Autodesk Fusion 360 part; units mm, degrees
(part 2 of 9)
  constraint tangent L185 A185
  constraint tangent L186 A185
  constraint equal A185 A186
  constraint tangent L186 A187
  constraint tangent L187 A187
  constraint equal A186 A187
  constraint horizontal L188
  constraint vertical L189
  constraint horizontal L190
  constraint vertical L191
  constraint tangent L188 A190
  constraint tangent L191 A190
  constraint tangent L188 A188
  constraint tangent L189 A188
  constraint equal A188 A190
  constraint tangent L189 A189
  constraint tangent L190 A189
  constraint equal A189 A190
  constraint tangent L190 A191
  constraint tangent L191 A191
  constraint equal A190 A191
  measures "d16" distance of L1 P0
  measures "d17" distance of L2 P0
  measures "d18" distance of P1 P2
  measures "d19" distance of P1 P3
  measures "d20" distance of P0 L11
  measures "d21" distance of P0 L8
  measures "d22" radius of A8
  measures "d23" distance of P0 P4
  measures "d24" radius of A13
  measures "d25" radius of A18
  measures "d26" radius of A22
  measures "d27" radius of A26
  measures "d28" radius of A30
  measures "d29" radius of A34
  measures "d30" radius of A38
  measures "d31" radius of A42
  measures "d32" radius of A46
  measures "d33" radius of A50
  measures "d34" radius of A54
  measures "d35" radius of A58
  measures "d36" radius of A62
  measures "d37" radius of A66
  measures "d38" radius of A70
  measures "d39" radius of A74
  measures "d40" radius of A78
  measures "d41" radius of A82
  measures "d42" radius of A86
  measures "d43" radius of A90
  measures "d44" radius of A94
  measures "d45" radius of A98
  measures "d46" radius of A102
  measures "d47" radius of A106
  measures "d48" radius of A110
  measures "d49" radius of A114
  measures "d50" radius of A118
  measures "d51" radius of A122
  measures "d52" radius of A126
  measures "d53" radius of A130
  measures "d54" radius of A134
  measures "d55" radius of A138
  measures "d56" radius of A142
  measures "d57" radius of A146
  measures "d58" radius of A150
  measures "d59" radius of A154
  measures "d60" radius of A158
  measures "d61" radius of A162
  measures "d62" radius of A166
  measures "d63" radius of A170
  measures "d64" radius of A174
  measures "d65" radius of A178
  measures "d66" radius of A182
  measures "d67" radius of A186
  measures "d68" radius of A190
extrude "Extrude3" cut sketch "Sketch3" against normal blind 5.1 contours L8 L9 L10 A9 A10 L188 L190 L191 A190 A191 | L9 A9 A10 L188 L189 L190 A188 A189 | A12 L12 A13 L13 A14 L14 L15 A15 | L16 L17 L18 L19 A16 A17 A18 A19 | L20 L21 L22 L23 A20 A21 A22 A23 | L24 L25 L26 L27 A24 A25 A26 A27 | L28 L29 L30 L31 A28 A29 A30 A31 | L32 L33 L34 L35 A32 A33 A34 A35 | L36 L37 L38 L39 A36 A37 A38 A39 | L40 L41 L42 L43 A40 A41 A42 A43 | L44 L45 L46 L47 A44 A45 A46 A47 | L48 L49 L50 L51 A48 A49 A50 A51 | L52 L53 L54 L55 A52 A53 A54 A55 | L56 L57 L58 L59 A56 A57 A58 A59 | L60 L61 L62 L63 A60 A61 A62 A63 | L64 L65 L66 L67 A64 A65 A66 A67 | L68 L69 L70 L71 A68 A69 A70 A71 | L72 L73 L74 L75 A72 A73 A74 A75 | L76 L77 L78 L79 A76 A77 A78 A79 | L80 L81 L82 L83 A80 A81 A82 A83 | L84 L85 L86 L87 A84 A85 A86 A87 | L88 L89 L90 L91 A88 A89 A90 A91 | L92 L93 L94 L95 A92 A93 A94 A95 | L96 L97 L98 L99 A96 A97 A98 A99 | L100 L101 L102 L103 A100 A101 A102 A103 | L104 L105 L106 L107 A104 A105 A106 A107 | L108 L109 L110 L111 A108 A109 A110 A111 | L112 L113 L114 L115 A112 A113 A114 A115 | L116 L117 L118 L119 A116 A117 A118 A119 | L120 L121 L122 L123 A120 A121 A122 A123 | L124 L125 L126 L127 A124 A125 A126 A127 | L128 L129 L130 L131 A128 A129 A130 A131 | L132 L133 L134 L135 A132 A133 A134 A135 | L136 L137 L138 L139 A136 A137 A138 A139 | L140 L141 L142 L143 A140 A141 A142 A143 | L144 L145 L146 L147 A144 A145 A146 A147 | L148 L149 L150 L151 A148 A149 A150 A151 | L152 L153 L154 L155 A152 A153 A154 A155 | L156 L157 L158 L159 A156 A157 A158 A159 | L160 L161 L162 L163 A160 A161 A162 A163 | L164 L165 L166 L167 A164 A165 A166 A167 | L168 L169 L170 L171 A168 A169 A170 A171 | L172 L173 L174 L175 A172 A173 A174 A175 | L176 L177 L178 L179 A176 A177 A178 A179 | L180 L181 L182 L183 A180 A181 A182 A183 | L184 L185 L186 L187 A184 A185 A186 A187
sketch "Sketch4" plane through (0, 5.1, 0) normal (0, 1, 0) x (-1, 0, 0)
  line L0 (-250.175, 15.525) -> (-250.175, 3.525)
  arc A0 (-251.175, 2.525) -> (-250.175, 3.525) centre (-251.175, 3.525) ccw
  line L1 (-251.175, 2.525) -> (-263.175, 2.525)
  arc A1 (-264.175, 3.525) -> (-263.175, 2.525) centre (-263.175, 3.525) ccw
  line L2 (-264.175, 3.525) -> (-264.175, 15.525)
  arc A2 (-263.175, 16.525) -> (-264.175, 15.525) centre (-263.175, 15.525) ccw
  line L3 (-263.175, 16.525) -> (-251.175, 16.525)
  arc A3 (-250.175, 15.525) -> (-251.175, 16.525) centre (-251.175, 15.525) ccw
  line L4 (-216.8375, 53.625) -> (-216.8375, 41.625)
  arc A4 (-217.8375, 40.625) -> (-216.8375, 41.625) centre (-217.8375, 41.625) ccw
  line L5 (-217.8375, 40.625) -> (-229.8375, 40.625)
  arc A5 (-230.8375, 41.625) -> (-229.8375, 40.625) centre (-229.8375, 41.625) ccw
  line L6 (-230.8375, 41.625) -> (-230.8375, 53.625)
  arc A6 (-229.8375, 54.625) -> (-230.8375, 53.625) centre (-229.8375, 53.625) ccw
  line L7 (-229.8375, 54.625) -> (-217.8375, 54.625)
  arc A7 (-216.8375, 53.625) -> (-217.8375, 54.625) centre (-217.8375, 53.625) ccw
  line L8 (-188.2625, 34.575) -> (-188.2625, 22.575)
  arc A8 (-189.2625, 21.575) -> (-188.2625, 22.575) centre (-189.2625, 22.575) ccw
  line L9 (-189.2625, 21.575) -> (-201.2625, 21.575)
  arc A9 (-202.2625, 22.575) -> (-201.2625, 21.575) centre (-201.2625, 22.575) ccw
  line L10 (-202.2625, 22.575) -> (-202.2625, 34.575)
  arc A10 (-201.2625, 35.575) -> (-202.2625, 34.575) centre (-201.2625, 34.575) ccw
  line L11 (-201.2625, 35.575) -> (-189.2625, 35.575)
  arc A11 (-188.2625, 34.575) -> (-189.2625, 35.575) centre (-189.2625, 34.575) ccw
  line L12 (-178.7375, 53.625) -> (-178.7375, 41.625)
  arc A12 (-179.7375, 40.625) -> (-178.7375, 41.625) centre (-179.7375, 41.625) ccw
  line L13 (-179.7375, 40.625) -> (-191.7375, 40.625)
  arc A13 (-192.7375, 41.625) -> (-191.7375, 40.625) centre (-191.7375, 41.625) ccw
  line L14 (-192.7375, 41.625) -> (-192.7375, 53.625)
  arc A14 (-191.7375, 54.625) -> (-192.7375, 53.625) centre (-191.7375, 53.625) ccw
  line L15 (-191.7375, 54.625) -> (-179.7375, 54.625)
  arc A15 (-178.7375, 53.625) -> (-179.7375, 54.625) centre (-179.7375, 53.625) ccw
  line L16 (-140.6375, 53.625) -> (-140.6375, 41.625)
  arc A16 (-141.6375, 40.625) -> (-140.6375, 41.625) centre (-141.6375, 41.625) ccw
  line L17 (-141.6375, 40.625) -> (-153.6375, 40.625)
  arc A17 (-154.6375, 41.625) -> (-153.6375, 40.625) centre (-153.6375, 41.625) ccw
  line L18 (-154.6375, 41.625) -> (-154.6375, 53.625)
  arc A18 (-153.6375, 54.625) -> (-154.6375, 53.625) centre (-153.6375, 53.625) ccw
  line L19 (-153.6375, 54.625) -> (-141.6375, 54.625)
  arc A19 (-140.6375, 53.625) -> (-141.6375, 54.625) centre (-141.6375, 53.625) ccw
  line L20 (-131.1125, 34.575) -> (-131.1125, 22.575)
  arc A20 (-132.1125, 21.575) -> (-131.1125, 22.575) centre (-132.1125, 22.575) ccw
  line L21 (-132.1125, 21.575) -> (-144.1125, 21.575)
  arc A21 (-145.1125, 22.575) -> (-144.1125, 21.575) centre (-144.1125, 22.575) ccw
  line L22 (-145.1125, 22.575) -> (-145.1125, 34.575)
  arc A22 (-144.1125, 35.575) -> (-145.1125, 34.575) centre (-144.1125, 34.575) ccw
  line L23 (-144.1125, 35.575) -> (-132.1125, 35.575)
  arc A23 (-131.1125, 34.575) -> (-132.1125, 35.575) centre (-132.1125, 34.575) ccw
  line L24 (-107.3, 15.525) -> (-107.3, 3.525)
  arc A24 (-108.3, 2.525) -> (-107.3, 3.525) centre (-108.3, 3.525) ccw
  line L25 (-108.3, 2.525) -> (-120.3, 2.525)
  arc A25 (-121.3, 3.525) -> (-120.3, 2.525) centre (-120.3, 3.525) ccw
  line L26 (-121.3, 3.525) -> (-121.3, 15.525)
  arc A26 (-120.3, 16.525) -> (-121.3, 15.525) centre (-120.3, 15.525) ccw
  line L27 (-120.3, 16.525) -> (-108.3, 16.525)
  arc A27 (-107.3, 15.525) -> (-108.3, 16.525) centre (-108.3, 15.525) ccw
  line L28 (-100.1562, 72.675) -> (-100.1562, 60.675)
  arc A28 (-101.1563, 59.675) -> (-100.1562, 60.675) centre (-101.1562, 60.675) ccw
  line L29 (-101.1563, 59.675) -> (-113.1562, 59.675)
  arc A29 (-114.1562, 60.675) -> (-113.1562, 59.675) centre (-113.1562, 60.675) ccw
  line L30 (-114.1562, 60.675) -> (-114.1562, 72.675)
  arc A30 (-113.1562, 73.675) -> (-114.1562, 72.675) centre (-113.1562, 72.675) ccw
  line L31 (-113.1562, 73.675) -> (-101.1562, 73.675)
  arc A31 (-100.1562, 72.675) -> (-101.1563, 73.675) centre (-101.1562, 72.675) ccw
  line L32 (-69.2, 15.525) -> (-69.2, 3.525)
  arc A32 (-70.2, 2.525) -> (-69.2, 3.525) centre (-70.2, 3.525) ccw
  line L33 (-70.2, 2.525) -> (-82.2, 2.525)
  arc A33 (-83.2, 3.525) -> (-82.2, 2.525) centre (-82.2, 3.525) ccw
  line L34 (-83.2, 3.525) -> (-83.2, 15.525)
  arc A34 (-82.2, 16.525) -> (-83.2, 15.525) centre (-82.2, 15.525) ccw
  line L35 (-82.2, 16.525) -> (-70.2, 16.525)
  arc A35 (-69.2, 15.525) -> (-70.2, 16.525) centre (-70.2, 15.525) ccw
  line L36 (-45.3875, 53.625) -> (-45.3875, 41.625)
  arc A36 (-46.3875, 40.625) -> (-45.3875, 41.625) centre (-46.3875, 41.625) ccw
  line L37 (-46.3875, 40.625) -> (-58.3875, 40.625)
  arc A37 (-59.3875, 41.625) -> (-58.3875, 40.625) centre (-58.3875, 41.625) ccw
  line L38 (-59.3875, 41.625) -> (-59.3875, 53.625)
  arc A38 (-58.3875, 54.625) -> (-59.3875, 53.625) centre (-58.3875, 53.625) ccw
  line L39 (-58.3875, 54.625) -> (-46.3875, 54.625)
  arc A39 (-45.3875, 53.625) -> (-46.3875, 54.625) centre (-46.3875, 53.625) ccw
  line L40 (-9.6688, 34.575) -> (-9.6687, 22.575)
  arc A40 (-10.6687, 21.575) -> (-9.6687, 22.575) centre (-10.6688, 22.575) ccw
  line L41 (-10.6687, 21.575) -> (-22.6688, 21.575)
  arc A41 (-23.6688, 22.575) -> (-22.6688, 21.575) centre (-22.6687, 22.575) ccw
  line L42 (-23.6688, 22.575) -> (-23.6687, 34.575)
  arc A42 (-22.6687, 35.575) -> (-23.6687, 34.575) centre (-22.6687, 34.575) ccw
  line L43 (-22.6688, 35.575) -> (-10.6688, 35.575)
  arc A43 (-9.6688, 34.575) -> (-10.6687, 35.575) centre (-10.6688, 34.575) ccw
  line L44 (-44.1, 16.525) -> (-32.1, 16.525)
  arc A44 (-31.1, 15.525) -> (-32.1, 16.525) centre (-32.1, 15.525) ccw
  line L45 (-31.1, 15.525) -> (-31.1, 3.525)
  arc A45 (-32.1, 2.525) -> (-31.1, 3.525) centre (-32.1, 3.525) ccw
  line L46 (-32.1, 2.525) -> (-44.1, 2.525)
  arc A46 (-45.1, 3.525) -> (-44.1, 2.525) centre (-44.1, 3.525) ccw
  line L47 (-45.1, 3.525) -> (-45.1, 15.525)
  arc A47 (-44.1, 16.525) -> (-45.1, 15.525) centre (-44.1, 15.525) ccw
  line L48 (-40.625, 72.675) -> (-40.625, 60.675)
  arc A48 (-41.625, 59.675) -> (-40.625, 60.675) centre (-41.625, 60.675) ccw
  line L49 (-41.625, 59.675) -> (-53.625, 59.675)
  arc A49 (-54.625, 60.675) -> (-53.625, 59.675) centre (-53.625, 60.675) ccw
  line L50 (-54.625, 60.675) -> (-54.625, 72.675)
  arc A50 (-53.625, 73.675) -> (-54.625, 72.675) centre (-53.625, 72.675) ccw
  line L51 (-53.625, 73.675) -> (-41.625, 73.675)
  arc A51 (-40.625, 72.675) -> (-41.625, 73.675) centre (-41.625, 72.675) ccw
  line L52 (-54.9125, 34.575) -> (-54.9125, 22.575)
  arc A52 (-55.9125, 21.575) -> (-54.9125, 22.575) centre (-55.9125, 22.575) ccw
  line L53 (-55.9125, 21.575) -> (-67.9125, 21.575)
  arc A53 (-68.9125, 22.575) -> (-67.9125, 21.575) centre (-67.9125, 22.575) ccw
  line L54 (-68.9125, 22.575) -> (-68.9125, 34.575)
  arc A54 (-67.9125, 35.575) -> (-68.9125, 34.575) centre (-67.9125, 34.575) ccw
  line L55 (-67.9125, 35.575) -> (-55.9125, 35.575)
  arc A55 (-54.9125, 34.575) -> (-55.9125, 35.575) centre (-55.9125, 34.575) ccw
  line L56 (-66.8188, 72.675) -> (-66.8188, 60.675)
  arc A56 (-67.8188, 59.675) -> (-66.8188, 60.675) centre (-67.8188, 60.675) ccw
  line L57 (-67.8188, 59.675) -> (-79.8188, 59.675)
  arc A57 (-80.8188, 60.675) -> (-79.8188, 59.675) centre (-79.8188, 60.675) ccw
  line L58 (-80.8187, 60.675) -> (-80.8187, 72.675)
  arc A58 (-79.8188, 73.675) -> (-80.8188, 72.675) centre (-79.8188, 72.675) ccw
  line L59 (-79.8188, 73.675) -> (-67.8188, 73.675)
  arc A59 (-66.8188, 72.675) -> (-67.8188, 73.675) centre (-67.8188, 72.675) ccw
  line L60 (-88.25, 15.525) -> (-88.25, 3.525)
  arc A60 (-89.25, 2.525) -> (-88.25, 3.525) centre (-89.25, 3.525) ccw
  line L61 (-89.25, 2.525) -> (-101.25, 2.525)
  arc A61 (-102.25, 3.525) -> (-101.25, 2.525) centre (-101.25, 3.525) ccw
  line L62 (-102.25, 3.525) -> (-102.25, 15.525)
  arc A62 (-101.25, 16.525) -> (-102.25, 15.525) centre (-101.25, 15.525) ccw
  line L63 (-101.25, 16.525) -> (-89.25, 16.525)
  arc A63 (-88.25, 15.525) -> (-89.25, 16.525) centre (-89.25, 15.525) ccw
  line L64 (-121.5875, 53.625) -> (-121.5875, 41.625)
  arc A64 (-122.5875, 40.625) -> (-121.5875, 41.625) centre (-122.5875, 41.625) ccw
  line L65 (-122.5875, 40.625) -> (-134.5875, 40.625)
  arc A65 (-135.5875, 41.625) -> (-134.5875, 40.625) centre (-134.5875, 41.625) ccw
  line L66 (-135.5875, 41.625) -> (-135.5875, 53.625)
  arc A66 (-134.5875, 54.625) -> (-135.5875, 53.625) centre (-134.5875, 53.625) ccw
  line L67 (-134.5875, 54.625) -> (-122.5875, 54.625)
  arc A67 (-121.5875, 53.625) -> (-122.5875, 54.625) centre (-122.5875, 53.625) ccw
  line L68 (-150.1625, 34.575) -> (-150.1625, 22.575)
  arc A68 (-151.1625, 21.575) -> (-150.1625, 22.575) centre (-151.1625, 22.575) ccw
  line L69 (-151.1625, 21.575) -> (-163.1625, 21.575)
  arc A69 (-164.1625, 22.575) -> (-163.1625, 21.575) centre (-163.1625, 22.575) ccw
  line L70 (-164.1625, 22.575) -> (-164.1625, 34.575)
  arc A70 (-163.1625, 35.575) -> (-164.1625, 34.575) centre (-163.1625, 34.575) ccw
  line L71 (-163.1625, 35.575) -> (-151.1625, 35.575)
  arc A71 (-150.1625, 34.575) -> (-151.1625, 35.575) centre (-151.1625, 34.575) ccw
  line L72 (-171.5938, 72.675) -> (-171.5937, 60.675)
  arc A72 (-172.5937, 59.675) -> (-171.5937, 60.675) centre (-172.5937, 60.675) ccw
  line L73 (-172.5938, 59.675) -> (-184.5938, 59.675)
  arc A73 (-185.5938, 60.675) -> (-184.5938, 59.675) centre (-184.5938, 60.675) ccw
  line L74 (-185.5938, 60.675) -> (-185.5937, 72.675)
  arc A74 (-184.5938, 73.675) -> (-185.5937, 72.675) centre (-184.5937, 72.675) ccw
  line L75 (-184.5938, 73.675) -> (-172.5937, 73.675)
  arc A75 (-171.5938, 72.675) -> (-172.5937, 73.675) centre (-172.5937, 72.675) ccw
  line L76 (-183.5, 15.525) -> (-183.5, 3.525)
  arc A76 (-184.5, 2.525) -> (-183.5, 3.525) centre (-184.5, 3.525) ccw
  line L77 (-184.5, 2.525) -> (-196.5, 2.525)
  arc A77 (-197.5, 3.525) -> (-196.5, 2.525) centre (-196.5, 3.525) ccw
  line L78 (-197.5, 3.525) -> (-197.5, 15.525)
  arc A78 (-196.5, 16.525) -> (-197.5, 15.525) centre (-196.5, 15.525) ccw
  line L79 (-196.5, 16.525) -> (-184.5, 16.525)
  arc A79 (-183.5, 15.525) -> (-184.5, 16.525) centre (-184.5, 15.525) ccw
  line L80 (-223.9813, 72.675) -> (-223.9813, 60.675)
  arc A80 (-224.9813, 59.675) -> (-223.9812, 60.675) centre (-224.9812, 60.675) ccw
  line L81 (-224.9813, 59.675) -> (-236.9813, 59.675)
  arc A81 (-237.9813, 60.675) -> (-236.9813, 59.675) centre (-236.9813, 60.675) ccw
  line L82 (-237.9813, 60.675) -> (-237.9812, 72.675)
  arc A82 (-236.9813, 73.675) -> (-237.9813, 72.675) centre (-236.9813, 72.675) ccw
  line L83 (-236.9813, 73.675) -> (-224.9813, 73.675)
  arc A83 (-223.9813, 72.675) -> (-224.9813, 73.675) centre (-224.9812, 72.675) ccw
  line L84 (-226.3625, 15.525) -> (-226.3625, 3.525)
  arc A84 (-227.3625, 2.525) -> (-226.3625, 3.525) centre (-227.3625, 3.525) ccw
  line L85 (-227.3625, 2.525) -> (-239.3625, 2.525)
  arc A85 (-240.3625, 3.525) -> (-239.3625, 2.525) centre (-239.3625, 3.525) ccw
  line L86 (-240.3625, 3.525) -> (-240.3625, 15.525)
  arc A86 (-239.3625, 16.525) -> (-240.3625, 15.525) centre (-239.3625, 15.525) ccw
  line L87 (-239.3625, 16.525) -> (-227.3625, 16.525)
  arc A87 (-226.3625, 15.525) -> (-227.3625, 16.525) centre (-227.3625, 15.525) ccw
  line L88 (-238.2688, 34.575) -> (-238.2688, 22.575)
  arc A88 (-239.2688, 21.575) -> (-238.2687, 22.575) centre (-239.2687, 22.575) ccw
  line L89 (-239.2688, 21.575) -> (-251.2688, 21.575)
  arc A89 (-252.2688, 22.575) -> (-251.2688, 21.575) centre (-251.2688, 22.575) ccw
  line L90 (-252.2688, 22.575) -> (-252.2688, 34.575)
  arc A90 (-251.2688, 35.575) -> (-252.2688, 34.575) centre (-251.2687, 34.575) ccw
  line L91 (-251.2688, 35.575) -> (-239.2688, 35.575)
  arc A91 (-238.2688, 34.575) -> (-239.2688, 35.575) centre (-239.2687, 34.575) ccw
  line L92 (-207.3125, 34.575) -> (-207.3125, 22.575)
  arc A92 (-208.3125, 21.575) -> (-207.3125, 22.575) centre (-208.3125, 22.575) ccw
  line L93 (-208.3125, 21.575) -> (-220.3125, 21.575)
  arc A93 (-221.3125, 22.575) -> (-220.3125, 21.575) centre (-220.3125, 22.575) ccw
  line L94 (-221.3125, 22.575) -> (-221.3125, 34.575)
  arc A94 (-220.3125, 35.575) -> (-221.3125, 34.575) centre (-220.3125, 34.575) ccw
  line L95 (-220.3125, 35.575) -> (-208.3125, 35.575)
  arc A95 (-207.3125, 34.575) -> (-208.3125, 35.575) centre (-208.3125, 34.575) ccw
  line L96 (-197.7875, 53.625) -> (-197.7875, 41.625)
  arc A96 (-198.7875, 40.625) -> (-197.7875, 41.625) centre (-198.7875, 41.625) ccw
  line L97 (-198.7875, 40.625) -> (-210.7875, 40.625)
  arc A97 (-211.7875, 41.625) -> (-210.7875, 40.625) centre (-210.7875, 41.625) ccw
  line L98 (-211.7875, 41.625) -> (-211.7875, 53.625)
  arc A98 (-210.7875, 54.625) -> (-211.7875, 53.625) centre (-210.7875, 53.625) ccw
  line L99 (-210.7875, 54.625) -> (-198.7875, 54.625)
  arc A99 (-197.7875, 53.625) -> (-198.7875, 54.625) centre (-198.7875, 53.625) ccw
  line L100 (-169.2125, 34.575) -> (-169.2125, 22.575)
  arc A100 (-170.2125, 21.575) -> (-169.2125, 22.575) centre (-170.2125, 22.575) ccw
  line L101 (-170.2125, 21.575) -> (-182.2125, 21.575)
  arc A101 (-183.2125, 22.575) -> (-182.2125, 21.575) centre (-182.2125, 22.575) ccw
  line L102 (-183.2125, 22.575) -> (-183.2125, 34.575)
  arc A102 (-182.2125, 35.575) -> (-183.2125, 34.575) centre (-182.2125, 34.575) ccw
  line L103 (-182.2125, 35.575) -> (-170.2125, 35.575)
  arc A103 (-169.2125, 34.575) -> (-170.2125, 35.575) centre (-170.2125, 34.575) ccw
  line L104 (-140.6375, 72.675) -> (-140.6375, 60.675)
  arc A104 (-141.6375, 59.675) -> (-140.6375, 60.675) centre (-141.6375, 60.675) ccw
  line L105 (-141.6375, 59.675) -> (-153.6375, 59.675)
  arc A105 (-154.6375, 60.675) -> (-153.6375, 59.675) centre (-153.6375, 60.675) ccw
  line L106 (-154.6375, 60.675) -> (-154.6375, 72.675)
  arc A106 (-153.6375, 73.675) -> (-154.6375, 72.675) centre (-153.6375, 72.675) ccw
  line L107 (-153.6375, 73.675) -> (-141.6375, 73.675)
  arc A107 (-140.6375, 72.675) -> (-141.6375, 73.675) centre (-141.6375, 72.675) ccw
  line L108 (-126.35, 15.525) -> (-126.35, 3.525)
  arc A108 (-127.35, 2.525) -> (-126.35, 3.525) centre (-127.35, 3.525) ccw
  line L109 (-127.35, 2.525) -> (-139.35, 2.525)
  arc A109 (-140.35, 3.525) -> (-139.35, 2.525) centre (-139.35, 3.525) ccw
  line L110 (-140.35, 3.525) -> (-140.35, 15.525)
  arc A110 (-139.35, 16.525) -> (-140.35, 15.525) centre (-139.35, 15.525) ccw
  line L111 (-139.35, 16.525) -> (-127.35, 16.525)
  arc A111 (-126.35, 15.525) -> (-127.35, 16.525) centre (-127.35, 15.525) ccw
  line L112 (-112.0625, 34.575) -> (-112.0625, 22.575)
  arc A112 (-113.0625, 21.575) -> (-112.0625, 22.575) centre (-113.0625, 22.575) ccw
  line L113 (-113.0625, 21.575) -> (-125.0625, 21.575)
  arc A113 (-126.0625, 22.575) -> (-125.0625, 21.575) centre (-125.0625, 22.575) ccw
  line L114 (-126.0625, 22.575) -> (-126.0625, 34.575)
  arc A114 (-125.0625, 35.575) -> (-126.0625, 34.575) centre (-125.0625, 34.575) ccw
  line L115 (-125.0625, 35.575) -> (-113.0625, 35.575)
  arc A115 (-112.0625, 34.575) -> (-113.0625, 35.575) centre (-113.0625, 34.575) ccw
  line L116 (-83.4875, 53.625) -> (-83.4875, 41.625)
  arc A116 (-84.4875, 40.625) -> (-83.4875, 41.625) centre (-84.4875, 41.625) ccw
  line L117 (-84.4875, 40.625) -> (-96.4875, 40.625)
  arc A117 (-97.4875, 41.625) -> (-96.4875, 40.625) centre (-96.4875, 41.625) ccw
  line L118 (-97.4875, 41.625) -> (-97.4875, 53.625)
  arc A118 (-96.4875, 54.625) -> (-97.4875, 53.625) centre (-96.4875, 53.625) ccw
  line L119 (-96.4875, 54.625) -> (-84.4875, 54.625)
  arc A119 (-83.4875, 53.625) -> (-84.4875, 54.625) centre (-84.4875, 53.625) ccw
  line L120 (-73.9625, 34.575) -> (-73.9625, 22.575)
  arc A120 (-74.9625, 21.575) -> (-73.9625, 22.575) centre (-74.9625, 22.575) ccw
  line L121 (-74.9625, 21.575) -> (-86.9625, 21.575)
  arc A121 (-87.9625, 22.575) -> (-86.9625, 21.575) centre (-86.9625, 22.575) ccw
  line L122 (-87.9625, 22.575) -> (-87.9625, 34.575)
  arc A122 (-86.9625, 35.575) -> (-87.9625, 34.575) centre (-86.9625, 34.575) ccw
  line L123 (-86.9625, 35.575) -> (-74.9625, 35.575)
  arc A123 (-73.9625, 34.575) -> (-74.9625, 35.575) centre (-74.9625, 34.575) ccw
  line L124 (-35.8625, 34.575) -> (-35.8625, 22.575)
  arc A124 (-36.8625, 21.575) -> (-35.8625, 22.575) centre (-36.8625, 22.575) ccw
  line L125 (-36.8625, 21.575) -> (-48.8625, 21.575)
  arc A125 (-49.8625, 22.575) -> (-48.8625, 21.575) centre (-48.8625, 22.575) ccw
  line L126 (-49.8625, 22.575) -> (-49.8625, 34.575)
  arc A126 (-48.8625, 35.575) -> (-49.8625, 34.575) centre (-48.8625, 34.575) ccw
  line L127 (-48.8625, 35.575) -> (-36.8625, 35.575)
  arc A127 (-35.8625, 34.575) -> (-36.8625, 35.575) centre (-36.8625, 34.575) ccw
  line L128 (-14.4313, 53.625) -> (-14.4313, 41.625)
  arc A128 (-15.4313, 40.625) -> (-14.4313, 41.625) centre (-15.4312, 41.625) ccw
  line L129 (-15.4313, 40.625) -> (-27.4313, 40.625)
  arc A129 (-28.4313, 41.625) -> (-27.4313, 40.625) centre (-27.4313, 41.625) ccw
  line L130 (-28.4313, 41.625) -> (-28.4313, 53.625)
  arc A130 (-27.4313, 54.625) -> (-28.4313, 53.625) centre (-27.4312, 53.625) ccw
  line L131 (-27.4313, 54.625) -> (-15.4313, 54.625)
  arc A131 (-14.4313, 53.625) -> (-15.4313, 54.625) centre (-15.4313, 53.625) ccw
  line L132 (-7.2875, 15.525) -> (-7.2875, 3.525)
  arc A132 (-8.2875, 2.525) -> (-7.2875, 3.525) centre (-8.2875, 3.525) ccw
  line L133 (-8.2875, 2.525) -> (-20.2875, 2.525)
  arc A133 (-21.2875, 3.525) -> (-20.2875, 2.525) centre (-20.2875, 3.525) ccw
  line L134 (-21.2875, 3.525) -> (-21.2875, 15.525)
  arc A134 (-20.2875, 16.525) -> (-21.2875, 15.525) centre (-20.2875, 15.525) ccw
  line L135 (-20.2875, 16.525) -> (-8.2875, 16.525)
  arc A135 (-7.2875, 15.525) -> (-8.2875, 16.525) centre (-8.2875, 15.525) ccw
  line L136 (-14.4313, 72.675) -> (-14.4313, 60.675)
  arc A136 (-15.4313, 59.675) -> (-14.4313, 60.675) centre (-15.4312, 60.675) ccw
  line L137 (-15.4313, 59.675) -> (-27.4313, 59.675)
  arc A137 (-28.4313, 60.675) -> (-27.4313, 59.675) centre (-27.4313, 60.675) ccw
  line L138 (-28.4313, 60.675) -> (-28.4312, 72.675)
  arc A138 (-27.4313, 73.675) -> (-28.4312, 72.675) centre (-27.4312, 72.675) ccw
  line L139 (-27.4313, 73.675) -> (-15.4313, 73.675)
  arc A139 (-14.4313, 72.675) -> (-15.4313, 73.675) centre (-15.4313, 72.675) ccw
  line L140 (-50.15, 15.525) -> (-50.15, 3.525)
  arc A140 (-51.15, 2.525) -> (-50.15, 3.525) centre (-51.15, 3.525) ccw
  line L141 (-51.15, 2.525) -> (-63.15, 2.525)
  arc A141 (-64.15, 3.525) -> (-63.15, 2.525) centre (-63.15, 3.525) ccw
  line L142 (-64.15, 3.525) -> (-64.15, 15.525)
  arc A142 (-63.15, 16.525) -> (-64.15, 15.525) centre (-63.15, 15.525) ccw
  line L143 (-63.15, 16.525) -> (-51.15, 16.525)
  arc A143 (-50.15, 15.525) -> (-51.15, 16.525) centre (-51.15, 15.525) ccw
  line L144 (-64.4375, 53.625) -> (-64.4375, 41.625)
  arc A144 (-65.4375, 40.625) -> (-64.4375, 41.625) centre (-65.4375, 41.625) ccw
  line L145 (-65.4375, 40.625) -> (-77.4375, 40.625)
  arc A145 (-78.4375, 41.625) -> (-77.4375, 40.625) centre (-77.4375, 41.625) ccw
  line L146 (-78.4375, 41.625) -> (-78.4375, 53.625)
  arc A146 (-77.4375, 54.625) -> (-78.4375, 53.625) centre (-77.4375, 53.625) ccw
  line L147 (-77.4375, 54.625) -> (-65.4375, 54.625)
  arc A147 (-64.4375, 53.625) -> (-65.4375, 54.625) centre (-65.4375, 53.625) ccw
  line L148 (-93.0125, 34.575) -> (-93.0125, 22.575)
  arc A148 (-94.0125, 21.575) -> (-93.0125, 22.575) centre (-94.0125, 22.575) ccw
  line L149 (-94.0125, 21.575) -> (-106.0125, 21.575)
  arc A149 (-107.0125, 22.575) -> (-106.0125, 21.575) centre (-106.0125, 22.575) ccw
  line L150 (-107.0125, 22.575) -> (-107.0125, 34.575)
  arc A150 (-106.0125, 35.575) -> (-107.0125, 34.575) centre (-106.0125, 34.575) ccw
  line L151 (-106.0125, 35.575) -> (-94.0125, 35.575)
  arc A151 (-93.0125, 34.575) -> (-94.0125, 35.575) centre (-94.0125, 34.575) ccw
  line L152 (-102.5375, 53.625) -> (-102.5375, 41.625)
  arc A152 (-103.5375, 40.625) -> (-102.5375, 41.625) centre (-103.5375, 41.625) ccw
  line L153 (-103.5375, 40.625) -> (-115.5375, 40.625)
  arc A153 (-116.5375, 41.625) -> (-115.5375, 40.625) centre (-115.5375, 41.625) ccw
  line L154 (-116.5375, 41.625) -> (-116.5375, 53.625)
  arc A154 (-115.5375, 54.625) -> (-116.5375, 53.625) centre (-115.5375, 53.625) ccw
  line L155 (-115.5375, 54.625) -> (-103.5375, 54.625)
  arc A155 (-102.5375, 53.625) -> (-103.5375, 54.625) centre (-103.5375, 53.625) ccw
  line L156 (-145.4, 15.525) -> (-145.4, 3.525)
  arc A156 (-146.4, 2.525) -> (-145.4, 3.525) centre (-146.4, 3.525) ccw
  line L157 (-146.4, 2.525) -> (-158.4, 2.525)
  arc A157 (-159.4, 3.525) -> (-158.4, 2.525) centre (-158.4, 3.525) ccw
  line L158 (-159.4, 3.525) -> (-159.4, 15.525)
  arc A158 (-158.4, 16.525) -> (-159.4, 15.525) centre (-158.4, 15.525) ccw
  line L159 (-158.4, 16.525) -> (-146.4, 16.525)
  arc A159 (-145.4, 15.525) -> (-146.4, 16.525) centre (-146.4, 15.525) ccw
  line L160 (-159.6875, 53.625) -> (-159.6875, 41.625)
  arc A160 (-160.6875, 40.625) -> (-159.6875, 41.625) centre (-160.6875, 41.625) ccw
  line L161 (-160.6875, 40.625) -> (-172.6875, 40.625)
  arc A161 (-173.6875, 41.625) -> (-172.6875, 40.625) centre (-172.6875, 41.625) ccw
  line L162 (-173.6875, 41.625) -> (-173.6875, 53.625)
  arc A162 (-172.6875, 54.625) -> (-173.6875, 53.625) centre (-172.6875, 53.625) ccw
  line L163 (-172.6875, 54.625) -> (-160.6875, 54.625)
  arc A163 (-159.6875, 53.625) -> (-160.6875, 54.625) centre (-160.6875, 53.625) ccw
  line L164 (-164.45, 15.525) -> (-164.45, 3.525)
  arc A164 (-165.45, 2.525) -> (-164.45, 3.525) centre (-165.45, 3.525) ccw
  line L165 (-165.45, 2.525) -> (-177.45, 2.525)
  arc A165 (-178.45, 3.525) -> (-177.45, 2.525) centre (-177.45, 3.525) ccw
  line L166 (-178.45, 3.525) -> (-178.45, 15.525)
  arc A166 (-177.45, 16.525) -> (-178.45, 15.525) centre (-177.45, 15.525) ccw
  line L167 (-177.45, 16.525) -> (-165.45, 16.525)
  arc A167 (-164.45, 15.525) -> (-165.45, 16.525) centre (-165.45, 15.525) ccw
  line L168 (-197.7875, 72.675) -> (-197.7875, 60.675)
  arc A168 (-198.7875, 59.675) -> (-197.7875, 60.675) centre (-198.7875, 60.675) ccw
  line L169 (-198.7875, 59.675) -> (-210.7875, 59.675)
  arc A169 (-211.7875, 60.675) -> (-210.7875, 59.675) centre (-210.7875, 60.675) ccw
  line L170 (-211.7875, 60.675) -> (-211.7875, 72.675)
  arc A170 (-210.7875, 73.675) -> (-211.7875, 72.675) centre (-210.7875, 72.675) ccw
  line L171 (-210.7875, 73.675) -> (-198.7875, 73.675)
  arc A171 (-197.7875, 72.675) -> (-198.7875, 73.675) centre (-198.7875, 72.675) ccw
  line L172 (-202.55, 15.525) -> (-202.55, 3.525)
  arc A172 (-203.55, 2.525) -> (-202.55, 3.525) centre (-203.55, 3.525) ccw
  line L173 (-203.55, 2.525) -> (-215.55, 2.525)
  arc A173 (-216.55, 3.525) -> (-215.55, 2.525) centre (-215.55, 3.525) ccw
  line L174 (-216.55, 3.525) -> (-216.55, 15.525)
  arc A174 (-215.55, 16.525) -> (-216.55, 15.525) centre (-215.55, 15.525) ccw
  line L175 (-215.55, 16.525) -> (-203.55, 16.525)
  arc A175 (-202.55, 15.525) -> (-203.55, 16.525) centre (-203.55, 15.525) ccw
  line L176 (-243.0312, 53.625) -> (-243.0312, 41.625)
  arc A176 (-244.0312, 40.625) -> (-243.0313, 41.625) centre (-244.0313, 41.625) ccw
  line L177 (-244.0312, 40.625) -> (-256.0312, 40.625)
  arc A177 (-257.0312, 41.625) -> (-256.0312, 40.625) centre (-256.0312, 41.625) ccw
  line L178 (-257.0312, 41.625) -> (-257.0312, 53.625)
  arc A178 (-256.0312, 54.625) -> (-257.0312, 53.625) centre (-256.0312, 53.625) ccw
  line L179 (-256.0312, 54.625) -> (-244.0312, 54.625)
  arc A179 (-243.0313, 53.625) -> (-244.0312, 54.625) centre (-244.0312, 53.625) ccw
  arc A180 (-263.7, 57.15) -> (-266.7, 54.15) centre (-263.7, 54.15) ccw
  line L180 (-266.7, 54.15) -> (-266.7, 3)
  arc A181 (-266.7, 3) -> (-263.7, 0) centre (-263.7, 3) ccw
  line L181 (-263.7, 0) -> (-3, 0)
  arc A182 (-3, 0) -> (0, 3) centre (-3, 3) ccw
  line L182 (0, 3) -> (0, 54.15)
  arc A183 (0, 54.15) -> (-3, 57.15) centre (-3, 54.15) ccw
  line L183 (-3, 57.15) -> (-8.525, 57.15)
  arc A184 (-9.525, 58.15) -> (-8.525, 57.15) centre (-8.525, 58.15) ccw
  line L184 (-9.525, 58.15) -> (-9.525, 73.2)
  arc A185 (-9.525, 73.2) -> (-12.525, 76.2) centre (-12.525, 73.2) ccw
  line L185 (-12.525, 76.2) -> (-239.8875, 76.2)
  arc A186 (-239.8875, 76.2) -> (-242.8875, 73.2) centre (-239.8875, 73.2) ccw
  line L186 (-242.8875, 73.2) -> (-242.8875, 58.15)
  arc A187 (-243.8875, 57.15) -> (-242.8875, 58.15) centre (-243.8875, 58.15) ccw
  line L187 (-243.8875, 57.15) -> (-263.7, 57.15)
  line L188 (-230.1688, 21.575) -> (-260.3688, 21.575)
  line L189 (-261.3688, 22.575) -> (-261.3688, 34.575)
  line L190 (-260.3688, 35.575) -> (-230.1688, 35.575)
  line L191 (-229.1688, 34.575) -> (-229.1688, 22.575)
  line L192 (-36.5313, 40.625) -> (-6.3312, 40.625)
  line L193 (-5.3312, 41.625) -> (-5.3313, 53.625)
  line L194 (-6.3313, 54.625) -> (-36.5312, 54.625)
  line L195 (-37.5312, 53.625) -> (-37.5312, 41.625)
  line L196 (-92.0563, 59.675) -> (-122.2563, 59.675)
  line L197 (-123.2563, 60.675) -> (-123.2563, 72.675)
  line L198 (-122.2563, 73.675) -> (-92.0563, 73.675)
  line L199 (-91.0563, 72.675) -> (-91.0563, 60.675)
  line L200 (-132.5375, 59.675) -> (-162.7375, 59.675)
  line L201 (-163.7375, 60.675) -> (-163.7375, 72.675)
  line L202 (-162.7375, 73.675) -> (-132.5375, 73.675)
  line L203 (-131.5375, 72.675) -> (-131.5375, 60.675)
  arc A188 (-92.0563, 59.675) -> (-91.0563, 60.675) centre (-92.0563, 60.675) ccw
  arc A189 (-91.0563, 72.675) -> (-92.0563, 73.675) centre (-92.0563, 72.675) ccw
  arc A190 (-122.2563, 73.675) -> (-123.2563, 72.675) centre (-122.2563, 72.675) ccw
  arc A191 (-123.2563, 60.675) -> (-122.2563, 59.675) centre (-122.2563, 60.675) ccw
  arc A192 (-132.5375, 59.675) -> (-131.5375, 60.675) centre (-132.5375, 60.675) ccw
  arc A193 (-131.5375, 72.675) -> (-132.5375, 73.675) centre (-132.5375, 72.675) ccw
  arc A194 (-162.7375, 73.675) -> (-163.7375, 72.675) centre (-162.7375, 72.675) ccw
  arc A195 (-163.7375, 60.675) -> (-162.7375, 59.675) centre (-162.7375, 60.675) ccw
  arc A196 (-230.1688, 21.575) -> (-229.1688, 22.575) centre (-230.1688, 22.575) ccw
  arc A197 (-229.1688, 34.575) -> (-230.1688, 35.575) centre (-230.1688, 34.575) ccw
  arc A198 (-261.3688, 22.575) -> (-260.3688, 21.575) centre (-260.3688, 22.575) ccw
  arc A199 (-260.3688, 35.575) -> (-261.3688, 34.575) centre (-260.3688, 34.575) ccw
  arc A200 (-37.5312, 41.625) -> (-36.5313, 40.625) centre (-36.5313, 41.625) ccw
  arc A201 (-36.5313, 54.625) -> (-37.5312, 53.625) centre (-36.5313, 53.625) ccw
  arc A202 (-5.3313, 53.625) -> (-6.3313, 54.625) centre (-6.3312, 53.625) ccw
  arc A203 (-6.3312, 40.625) -> (-5.3312, 41.625) centre (-6.3312, 41.625) ccw
  point P0 (-21.4313, 47.625)
  point P1 (-107.1563, 66.675)
  point P2 (-147.6375, 66.675)
  point P3 (-245.2688, 28.575)
  point P4 (-229.1688, 21.575)
  point P5 (-261.3688, 21.575)
  point P6 (-37.5313, 40.625)
  point P7 (-5.3313, 40.625)
  point P8 (-91.0563, 59.675)
  point P9 (-123.2563, 59.675)
  point P10 (-131.5375, 59.675)
  point P11 (-163.7375, 59.675)
  dimension "d71" = 32.2
  dimension "d72" = 16.1
  dimension "d73" = 32.2
  dimension "d74" = 16.1
  dimension "d75" = 32.2
  dimension "d76" = 32.2
  dimension "d77" = 16.1
  dimension "d78" = 16.1
  dimension "d79" = 1
  constraint horizontal L188
  constraint vertical L189
  constraint horizontal L190
  constraint vertical L191
  constraint coincident L89 P4
  constraint horizontal L192
  constraint vertical L193
  constraint horizontal L194
  constraint vertical L195
  constraint coincident L129 P6
  constraint horizontal L196
  constraint vertical L197
  constraint horizontal L198
  constraint vertical L199
  constraint coincident L29 P8
  constraint horizontal L200
  constraint vertical L201
  constraint horizontal L202
  constraint vertical L203
  constraint coincident L105 P10
  constraint coincident P8 L196
  constraint coincident P8 L199
  constraint tangent L196 A188
  constraint tangent L199 A188
  constraint tangent L198 A189
  constraint tangent L199 A189
  constraint equal A188 A189
  constraint tangent L197 A190
  constraint tangent L198 A190
  constraint equal A188 A190
  constraint coincident P9 L196
  constraint coincident P9 L197
  constraint tangent L196 A191
  constraint tangent L197 A191
  constraint equal A188 A191
  constraint coincident P10 L200
  constraint coincident P10 L203
  constraint tangent L200 A192
  constraint tangent L203 A192
  constraint equal A188 A192
  constraint tangent L202 A193
  constraint tangent L203 A193
  constraint equal A188 A193
  constraint tangent L201 A194
  constraint tangent L202 A194
  constraint equal A188 A194
  constraint coincident P11 L200
  constraint coincident P11 L201
  constraint tangent L200 A195
  constraint tangent L201 A195
  constraint equal A188 A195
  constraint coincident P4 L188
  constraint coincident P4 L191
  constraint tangent L188 A196
  constraint tangent L191 A196
  constraint equal A188 A196
  constraint tangent L190 A197
  constraint tangent L191 A197
  constraint equal A188 A197
  constraint coincident P5 L188
  constraint coincident P5 L189
  constraint tangent L188 A198
  constraint tangent L189 A198
  constraint equal A188 A198
  constraint tangent L189 A199
  constraint tangent L190 A199
  constraint equal A188 A199
  constraint coincident P6 L192
  constraint coincident P6 L195
  constraint tangent L192 A200
  constraint tangent L195 A200
  constraint equal A188 A200
  constraint tangent L194 A201
  constraint tangent L195 A201
  constraint equal A188 A201
  constraint tangent L193 A202
  constraint tangent L194 A202
  constraint equal A188 A202
  constraint coincident P7 L192
  constraint coincident P7 L193
  constraint tangent L192 A203
  constraint tangent L193 A203
  constraint equal A188 A203
  measures "d71" distance of P4 P5
  measures "d72" distance of P3 L191
  measures "d73" distance of P6 P7
  measures "d74" distance of P0 L195
  measures "d75" distance of P8 P9
  measures "d76" distance of P10 P11
  measures "d77" distance of P2 L203
  measures "d78" distance of P1 L199
  measures "d79" radius of A188
extrude "Extrude4" cut sketch "Sketch4" against normal blind 5.1 contours L28 A28 A31 L196 L198 L199 A188 A189 | A29 L30 A30 L196 L197 L198 A190 A191 | L88 A88 A91 L188 L190 L191 A196 A197 | A89 L90 A90 L188 L189 L190 A198 A199 | L104 A104 A107 L200 L202 L203 A192 A193 | A105 L106 A106 L200 L201 L202 A194 A195 | L128 A128 A131 L192 L193 L194 A202 A203 | A129 L130 A130 L192 L194 L195 A200 A201